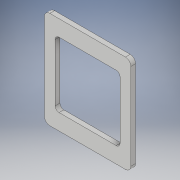
# Autodesk Inventor part: ESC Hole Test
Saved by Autodesk Inventor 2017.3 (Build 213256000, 256)
## iProperties
Created: 2019-01-11
Part Number: ESC Hole Test
Material: Generic
Document SubType Name: Modeling
Designer: LSabe
Density: 1 g/cm^3
Appearance: Default
Author: LSabe
Autodesk Inventor part; units mm, degrees
ref_plane "YZ Plane" through (0, 0, 0) normal (1, 0, 0) x (0, 1, 0)
ref_plane "XZ Plane" through (0, 0, 0) normal (0, 1, 0) x (-1, 0, 0)
ref_plane "XY Plane" through (0, 0, 0) normal (0, 0, 1) x (1, 0, 0)
sketch "Sketch1" plane through (0, 0, 0) normal (0, 0, 1) x (1, 0, 0)
  line L0 (0, 19.177) -> (19.0817, 19.177)
  line L1 (-6.3183, -9.398) -> (44.4817, -9.398)
  line L2 (44.4817, -9.398) -> (44.4817, 47.752)
  line L3 (44.4817, 47.752) -> (-6.3183, 47.752)
  line L4 (-6.3183, 47.752) -> (-6.3183, -9.398)
  line L5 (-6.3183, -9.398) -> (44.4817, 47.752) construction
  line L6 (44.4817, -9.398) -> (-6.3183, 47.752) construction
  line L7 (2.305, 0) -> (35.8584, 0)
  line L8 (38.1444, 2.286) -> (38.1444, 36.068)
  line L9 (35.8584, 38.354) -> (2.305, 38.354)
  line L10 (0.019, 36.068) -> (0.019, 2.286)
  line L11 (0.019, 0) -> (38.1444, 38.354) construction
  line L12 (38.1444, 0) -> (0.019, 38.354) construction
  arc A0 (2.305, 38.354) -> (0.019, 36.068) centre (2.305, 36.068) ccw
  arc A1 (38.1444, 36.068) -> (35.8584, 38.354) centre (35.8584, 36.068) ccw
  arc A2 (35.8584, 0) -> (38.1444, 2.286) centre (35.8584, 2.286) ccw
  arc A3 (0.019, 2.286) -> (2.305, 0) centre (2.305, 2.286) ccw
  dimension "d15" = 50.8
  dimension "d16" = 57.15
  dimension "d19" = 38.1254
  dimension "d20" = 38.354
  dimension "d21" = 2.286
  constraints: 26 end point, 8 point on circle, 8 point on line, 8 tangent, 4 centre point, 4 midpoint, 4 parallel, 3 equal radius, 3 horizontal, 2 perpendicular
  measures "d15" distance of L3.end L2.end
  measures "d16" distance of L2.end L1.end
  measures "d19" distance of L12.end L11.end
  measures "d20" distance of L11.end L12.start
  measures "d21" radius of A0
extrude "Extrusion1" add sketch "Sketch1" along normal blind 2.794
fillet "Fillet4" radius 3.175 4 edges at (-6.3183, 47.752, 1.397) (44.4817, 47.752, 1.397) (44.4817, -9.398, 1.397) (-6.3183, -9.398, 1.397)
body "Solid1"
